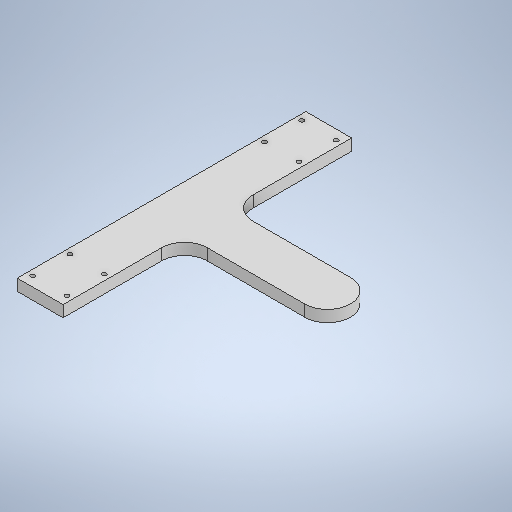
# Autodesk Inventor part: Chassis Rear Spine
Saved by Autodesk Inventor 2025.2 (Build 292293000, 293)
## iProperties
Created: 2025-02-18
Part Number: Chassis Rear Spine
Material: Generic
Document SubType Name: Modeling
Designer: mtidd
Density: 1 g/cm^3
Appearance: Default
Author: mtidd
Autodesk Inventor part; units mm, degrees
ref_plane "YZ Plane" through (0, 0, 0) normal (1, 0, 0) x (0, 1, 0)
ref_plane "XZ Plane" through (0, 0, 0) normal (0, 1, 0) x (-1, 0, 0)
ref_plane "XY Plane" through (0, 0, 0) normal (0, 0, 1) x (1, 0, 0)
sketch "Sketch1" plane through (0, 0, 0) normal (0, 1, 0) x (-1, 0, 0)
  line L0 (0, 0) -> (40, 0)
  line L1 (40, 0) -> (40, -126)
  line L2 (40, -126) -> (0, -126)
  line L3 (0, -126) -> (0, 0)
  line L4 (40, 0) -> (0, 0)
  line L5 (0, 0) -> (0, 126)
  line L6 (0, 126) -> (40, 126)
  line L7 (40, 126) -> (40, 0)
  line L8 (0, 0) -> (-125, 0)
  line L9 (-125, 0) -> (-125, -20)
  line L10 (-125, -20) -> (0, -20)
  line L11 (0, -20) -> (0, 0)
  line L12 (-125, -20) -> (0, -20)
  line L13 (0, -20) -> (0, 20)
  line L14 (0, 20) -> (-125, 20)
  line L15 (-125, 20) -> (-125, -20)
  line L16 (35, -126) -> (35, 126) construction
  line L17 (40, -117.5) -> (0, -117.5) construction
  line L18 (40, 117.5) -> (0, 117.5) construction
  line L19 (20, 126) -> (20, -126) construction
  line L20 (5, -126) -> (5, 126) construction
  circle A0 centre (35, 117.5) radius 1.8
  circle A1 centre (5, 117.5) radius 1.8
  circle A2 centre (35, -117.5) radius 1.8
  circle A3 centre (5, -117.5) radius 1.8
  circle A4 centre (35, -85) radius 1.8
  circle A5 centre (5, -85) radius 1.8
  line L21 (35, 117.5) -> (5, 117.5) construction
  line L22 (5, 117.5) -> (5, 85) construction
  line L23 (5, 85) -> (35, 85) construction
  line L24 (35, 85) -> (35, 117.5) construction
  circle A6 centre (35, 85) radius 1.8
  circle A7 centre (5, 85) radius 1.8
  dimension "d0" = 40
  dimension "d1" = 126
  dimension "d2" = 40
  dimension "d3" = 126
  dimension "d4" = 125
  dimension "d5" = 20
  dimension "d6" = 125
  dimension "d7" = 40
  dimension "d8" = 3.6
  dimension "d9" = 3.6
  dimension "d10" = 3.6
  dimension "d11" = 3.6
  dimension "d12" = 3.6
  dimension "d13" = 3.6
  dimension "d14" = 30
  dimension "d15" = 32.5
  dimension "d16" = 3.6
  dimension "d17" = 3.6
  constraints: 50 end point, 14 point on line, 10 parallel, 8 centre point, 7 perpendicular, 5 horizontal, 4 symmetric about line, 2 coincident, 2 midpoint
  measures "d0" distance of L1.end L2.end
  measures "d1" distance of L0.end L1.end
  measures "d2" distance of L5.end L6.end
  measures "d3" distance of L4.end L5.end
  measures "d4" distance of L10.end L9.end
  measures "d5" distance of L9.end L8.end
  measures "d6" distance of L14.end L13.end
  measures "d7" distance of L13.end L12.end
  measures "d8" diameter of A0
  measures "d9" diameter of A1
  measures "d10" diameter of A2
  measures "d11" diameter of A3
  measures "d12" diameter of A4
  measures "d13" diameter of A5
  measures "d14" distance of L23.end L22.end
  measures "d15" distance of L22.end L21.end
  measures "d16" diameter of A6
  measures "d17" diameter of A7
extrude "Extrusion1" add sketch "Sketch1" along normal blind 10
fillet "Fillet1" radius 20 4 edges at (0, 5, 20) (0, 5, -20) (125, 5, -20) (125, 5, 20)
body "Solid1"
